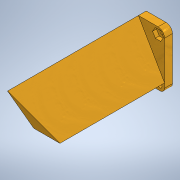
# Autodesk Inventor part: Doigt droit
Saved by Autodesk Inventor 2022 (Build 260153000, 153)
## iProperties
Created: 2022-04-30
Part Number: Doigt droit
Material: Générique
Document SubType Name: Modeling
Designer: victo
Density: 1 g/cm^3
Appearance: Soudure - Laiton
Author: victo
Autodesk Inventor part; units mm, degrees
ref_plane "YZ Plane" through (0, 0, 0) normal (1, 0, 0) x (0, 1, 0)
ref_plane "XZ Plane" through (0, 0, 0) normal (0, 1, 0) x (-1, 0, 0)
ref_plane "XY Plane" through (0, 0, 0) normal (0, 0, 1) x (1, 0, 0)
sketch "Esquisse1" plane through (0, 0, 0) normal (0, 0, 1) x (1, 0, 0)
  line L0 (0, 0) -> (-20, 34.641)
  line L1 (-20, 34.641) -> (-20, 0)
  line L2 (-20, 0) -> (0, 0)
  line L3 (-20, 34.641) -> (0, 34.641)
  line L4 (0, 34.641) -> (0, 0)
  circle A0 centre (-5, 29.641) radius 5
  circle A1 centre (-5, 29.641) radius 1.55
  line L5 (-7.0785, 26.041) -> (-9.1569, 29.641)
  line L6 (-9.1569, 29.641) -> (-7.0785, 33.241)
  line L7 (-7.0785, 33.241) -> (-2.9215, 33.241)
  line L8 (-2.9215, 33.241) -> (-0.8431, 29.641)
  line L9 (-0.8431, 29.641) -> (-2.9215, 26.041)
  line L10 (-2.9215, 26.041) -> (-7.0785, 26.041)
  line L11 (-20, 0) -> (-20, -7)
  line L12 (-20, -7) -> (0, -7)
  line L13 (0, -7) -> (0, 0)
  line L14 (-20, -3.5) -> (0, -3.5)
  circle A2 centre (-16.5, -3.5) radius 3.5
  circle A3 centre (-3.5, -3.5) radius 3.5
  circle A4 centre (-16.5, -3.5) radius 1.55
  circle A5 centre (-3.5, -3.5) radius 1.55
  point P0 (-16.5, -7)
  point P1 (-3.5, -7)
  point P2 (0, 29.641)
  point P3 (-5, 34.641)
  dimension "d0" = 60
  dimension "d1" = 20
  dimension "d5" = 7
  dimension "d6" = 3.1
  dimension "d7" = 10
  dimension "d8" = 7.2
  dimension "d9" = 3.1
  constraints: 30 end point, 4 centre point, 4 coincident, 4 perpendicular, 3 horizontal, 2 midpoint, 2 point on line, 2 tangent, 2 vertical, 1 equal radius, 19 other
  measures "d0" angle of L2 L0
  measures "d1" distance of L0.start L1.end
  measures "d5" distance between parallel lines of L12 L2
  measures "d6" diameter of A4
  measures "d7" diameter of A0
  measures "d8" distance between parallel lines of L10 L7
  measures "d9" diameter of A1
extrude "Extrusion1" add sketch "Esquisse1" along normal blind 100 contours L2 L1 L0
extrude "Extrusion2" add sketch "Esquisse1" against normal blind 6 contours L2 L1 L0 | L13 A3 L2 | L0 L3 A0 L4 | A3 L14 A2 L2 | A3 L14 A5 | A0 | A3 L14 A5 | L2 A2 L11 | A2 L14 A4 | A3 L12 A2 L14 | L14 A4 A2 | L5 L6 L7 L8 L9 L10
extrude "Extrusion3" cut sketch "Esquisse1" against normal blind 3 contours L5 L6 L7 L8 L9 L10
sketch "Esquisse2" plane through (0, 0, 0) normal (1, 0, 0) x (0, 0, -1)
  line L0 (-100, 34.641) -> (-100, 0) projected
  line L1 (-100, 34.641) -> (-80, 0)
  line L2 (0, 0) -> (-100, 0) projected
  line L3 (-80, 0) -> (-100, 0)
  line L4 (-100, 0) -> (-100, 34.641)
  dimension "d16" = 30
  constraints: 6 end point, 1 collinear, 1 perpendicular
  measures "d16" angle of L0 L1
extrude "Extrusion4" cut sketch "Esquisse2" against normal through all
